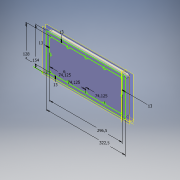
# Autodesk Inventor part: Крыша2
Saved by Autodesk Inventor 2018.3 (Build 223284000, 284)
## iProperties
Created: 2018-05-19
Part Number: Крыша2
Material: Типовые
Document SubType Name: Modeling
Designer: kriku
Density: 1 g/cm^3
Appearance: По умолчанию
Mass: 394.058 g
Surface Area: 1257.57 cm^2
Volume: 394.058 cm^3
Author: kriku
Autodesk Inventor part; units mm, degrees
sketch "Эскиз1" plane through (0, 0, 0) normal (0, 1, 0) x (-1, 0, 0)
  arc A0 (294.6508, 19) -> (288.6508, 13) centre (294.6508, 13) ccw
  arc A1 (226.5258, 13) -> (214.5258, 13) centre (220.5258, 13) ccw
  arc A2 (152.4008, 13) -> (140.4008, 13) centre (146.4008, 13) ccw
  arc A3 (4.1508, 13) -> (-1.8492, 19) centre (-1.8492, 13) ccw
  arc A4 (78.2758, 13) -> (66.2758, 13) centre (72.2758, 13) ccw
  arc A5 (294.6508, 83) -> (294.6508, 71) centre (294.6508, 77) ccw
  arc A6 (288.6508, 141) -> (294.6508, 135) centre (294.6508, 141) ccw
  arc A7 (214.5258, 141) -> (226.5258, 141) centre (220.5258, 141) ccw
  arc A8 (140.4008, 141) -> (152.4008, 141) centre (146.4008, 141) ccw
  arc A9 (66.2758, 141) -> (78.2758, 141) centre (72.2758, 141) ccw
  arc A10 (-1.8492, 135) -> (4.1508, 141) centre (-1.8492, 141) ccw
  arc A11 (-1.8492, 71) -> (-1.8492, 83) centre (-1.8492, 77) ccw
  line L0 (-14.8492, 10.5) -> (-14.8492, 143.5)
  line L1 (-14.8492, 10.5) -> (-14.8492, 143.5)
  line L2 (-4.3492, 154) -> (297.1508, 154)
  line L3 (307.6508, 10.5) -> (307.6508, 143.5)
  line L4 (297.1508, 0) -> (-4.3492, 0)
  line L5 (288.6508, 13) -> (226.5258, 13)
  line L6 (214.5258, 13) -> (152.4008, 13)
  line L7 (140.4008, 13) -> (78.2758, 13)
  line L8 (66.2758, 13) -> (4.1508, 13)
  line L9 (-1.8492, 19) -> (-1.8492, 71)
  line L10 (-1.8492, 83) -> (-1.8492, 135)
  line L11 (4.1508, 141) -> (66.2758, 141)
  line L12 (78.2758, 141) -> (140.4008, 141)
  line L13 (152.4008, 141) -> (214.5258, 141)
  line L14 (226.5258, 141) -> (288.6508, 141)
  line L15 (294.6508, 135) -> (294.6508, 83)
  line L16 (294.6508, 71) -> (294.6508, 19)
  line L17 (275.1508, 0) -> (362.1508, 0)
  line L18 (307.6508, 0) -> (-14.8492, 0)
  line L19 (-14.8492, 0) -> (-14.8492, 154)
  line L20 (-14.8492, 154) -> (307.6508, 154)
  line L21 (307.6508, 154) -> (307.6508, 0)
  point P0 (0, 0)
  point P1 (323.6508, -3)
  point P2 (297.1508, 10.5)
  point P3 (-4.3492, 10.5)
  point P4 (-4.3492, 143.5)
  point P5 (146.4008, 13)
  dimension "d0" = 74.125
  dimension "d1" = 74.125
  dimension "d2" = 74.125
  dimension "d3" = 6
  dimension "d4" = 296.5
  dimension "d5" = 322.5
  dimension "d6" = 154
  dimension "d7" = 128
  dimension "d8" = 13
  dimension "d9" = 13
  dimension "d10" = 13
  dimension "d11" = 13
  constraints: 44 end point, 27 point on circle, 14 coincident, 12 centre point, 11 equal radius, 4 equal length, 2 vertical alignment, 1 horizontal, 1 horizontal alignment, 1 perpendicular, 1 point on line
  measures "d0" distance of point (220.526, 13) point (294.651, 13)
  measures "d1" distance of point (220.526, 13) point (146.401, 13)
  measures "d2" distance of point (72.276, 13) point (146.401, 13)
  measures "d3" radius of A1
  measures "d4" distance between parallel lines of L10 L15
  measures "d5" distance between parallel lines of L19 L3
  measures "d6" distance between parallel lines of L18 L20
  measures "d7" distance between parallel lines of L5 L14
  measures "d8" distance between parallel lines of L19 L10
  measures "d9" distance between parallel lines of L21 L15
  measures "d10" distance between parallel lines of L18 L5
  measures "d11" distance between parallel lines of L2 L14
extrude "Выдавливание1" add sketch "Эскиз1" along normal blind 17
extrude "Выдавливание2" add sketch "Эскиз1" along normal blind 5 contours A0 L5 A1 L6 A2 L7 A4 L8 A3 L9 A11 L10 A10 L11 A9 L12 A8 L13 A7 L14 A6 L15 A5 L16 | L0 L19 L20 L2 L21 L3 L17 L4 L18
fillet "Сопряжение1" radius 10.5 4 edges at (-307.6508, 8.5, 0) (14.8492, 8.5, 0) (-307.6508, 8.5, 154) (14.8492, 8.5, 154)
ref_plane "РабПлоскость1" through (0, 14.5, 0) normal (0, 1, 0) x (1, 0, 0)
sketch "Эскиз5" plane through (0, 5, 0) normal (0, 1, 0) x (1, 0, 0)
  line L0 (-140.4008, -13) -> (-78.2758, -13) projected
  arc A0 (-152.4008, -13) -> (-140.4008, -13) centre (-146.4008, -13) ccw projected
  line L1 (-214.5258, -13) -> (-152.4008, -13) projected
  arc A1 (-226.5258, -13) -> (-214.5258, -13) centre (-220.5258, -13) ccw projected
  line L2 (-288.6508, -13) -> (-226.5258, -13) projected
  arc A2 (-294.6508, -19) -> (-288.6508, -13) centre (-294.6508, -13) ccw projected
  line L3 (-294.6508, -71) -> (-294.6508, -19) projected
  arc A3 (-294.6508, -83) -> (-294.6508, -71) centre (-294.6508, -77) ccw projected
  line L4 (-294.6508, -135) -> (-294.6508, -83) projected
  arc A4 (-288.6508, -141) -> (-294.6508, -135) centre (-294.6508, -141) ccw projected
  line L5 (-226.5258, -141) -> (-288.6508, -141) projected
  arc A5 (-214.5258, -141) -> (-226.5258, -141) centre (-220.5258, -141) ccw projected
  line L6 (-152.4008, -141) -> (-214.5258, -141) projected
  arc A6 (-140.4008, -141) -> (-152.4008, -141) centre (-146.4008, -141) ccw projected
  line L7 (-78.2758, -141) -> (-140.4008, -141) projected
  arc A7 (-66.2758, -141) -> (-78.2758, -141) centre (-72.2758, -141) ccw projected
  line L8 (-4.1508, -141) -> (-66.2758, -141) projected
  arc A8 (1.8492, -135) -> (-4.1508, -141) centre (1.8492, -141) ccw projected
  line L9 (1.8492, -83) -> (1.8492, -135) projected
  arc A9 (1.8492, -71) -> (1.8492, -83) centre (1.8492, -77) ccw projected
  line L10 (1.8492, -19) -> (1.8492, -71) projected
  arc A10 (-4.1508, -13) -> (1.8492, -19) centre (1.8492, -13) ccw projected
  line L11 (-66.2758, -13) -> (-4.1508, -13) projected
  arc A11 (-78.2758, -13) -> (-66.2758, -13) centre (-72.2758, -13) ccw projected
  point P0 (0, 0)
sketch "Эскиз4" plane through (0, 14.5, 0) normal (0, 1, 0) x (1, 0, 0)
  line L0 (-140.4008, -13) -> (-78.2758, -13) projected
  arc A0 (-78.2758, -13) -> (-66.2758, -13) centre (-72.2758, -13) ccw projected
  line L1 (-66.2758, -13) -> (-4.1508, -13) projected
  arc A1 (-4.1508, -13) -> (1.8492, -19) centre (1.8492, -13) ccw projected
  line L2 (1.8492, -19) -> (1.8492, -71) projected
  arc A2 (1.8492, -71) -> (1.8492, -83) centre (1.8492, -77) ccw projected
  line L3 (1.8492, -83) -> (1.8492, -135) projected
  arc A3 (1.8492, -135) -> (-4.1508, -141) centre (1.8492, -141) ccw projected
  line L4 (-4.1508, -141) -> (-66.2758, -141) projected
  arc A4 (-66.2758, -141) -> (-78.2758, -141) centre (-72.2758, -141) ccw projected
  line L5 (-78.2758, -141) -> (-140.4008, -141) projected
  arc A5 (-140.4008, -141) -> (-152.4008, -141) centre (-146.4008, -141) ccw projected
  line L6 (-152.4008, -141) -> (-214.5258, -141) projected
  arc A6 (-214.5258, -141) -> (-226.5258, -141) centre (-220.5258, -141) ccw projected
  line L7 (-226.5258, -141) -> (-288.6508, -141) projected
  arc A7 (-288.6508, -141) -> (-294.6508, -135) centre (-294.6508, -141) ccw projected
  line L8 (-294.6508, -135) -> (-294.6508, -83) projected
  arc A8 (-294.6508, -83) -> (-294.6508, -71) centre (-294.6508, -77) ccw projected
  line L9 (-294.6508, -71) -> (-294.6508, -19) projected
  arc A9 (-294.6508, -19) -> (-288.6508, -13) centre (-294.6508, -13) ccw projected
  line L10 (-288.6508, -13) -> (-226.5258, -13) projected
  arc A10 (-226.5258, -13) -> (-214.5258, -13) centre (-220.5258, -13) ccw projected
  line L11 (-214.5258, -13) -> (-152.4008, -13) projected
  arc A11 (-152.4008, -13) -> (-140.4008, -13) centre (-146.4008, -13) ccw projected
  arc A12 (4.3492, -154) -> (14.8492, -143.5) centre (4.3492, -143.5) ccw projected
  line L12 (14.8492, -143.5) -> (14.8492, -10.5) projected
  arc A13 (14.8492, -10.5) -> (4.3492, 0) centre (4.3492, -10.5) ccw projected
  line L13 (4.3492, 0) -> (-297.1508, 0) projected
  arc A14 (-297.1508, 0) -> (-307.6508, -10.5) centre (-297.1508, -10.5) ccw projected
  line L14 (-307.6508, -10.5) -> (-307.6508, -143.5) projected
  arc A15 (-307.6508, -143.5) -> (-297.1508, -154) centre (-297.1508, -143.5) ccw projected
  line L15 (-297.1508, -154) -> (4.3492, -154) projected
  arc A16 (-226.5258, -13) -> (-214.5258, -13) centre (-220.5258, -13) ccw projected
  line L16 (-220.5258, -13) -> (-220.5258, -141)
  line L17 (-146.4008, -13) -> (-146.4008, -141)
  line L18 (-72.2758, -13) -> (-72.2758, -141)
  line L19 (-294.6508, -77) -> (1.8492, -77)
  point P0 (0, 0)
  constraints: 8 end point, 2 vertical, 1 horizontal, 1 perpendicular
